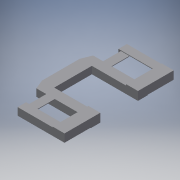
# Autodesk Inventor part: battlebotupperframe
Saved by Autodesk Inventor 2019 (Build 230136000, 136)
## iProperties
Created: 2018-08-05
Part Number: battlebotupperframe
Material: Generic
Document SubType Name: Modeling
Designer: Kitte_X
Density: 1 g/cm^3
Appearance: Default
Author: Kitte_X
Autodesk Inventor part; units mm, degrees
ref_plane "YZ Plane" through (0, 0, 0) normal (1, 0, 0) x (0, 1, 0)
ref_plane "XZ Plane" through (0, 0, 0) normal (0, 1, 0) x (-1, 0, 0)
ref_plane "XY Plane" through (0, 0, 0) normal (0, 0, 1) x (1, 0, 0)
sketch "Sketch1" plane through (0, 0, 0) normal (0, 1, 0) x (-1, 0, 0)
  line L0 (-100, 284.5) -> (-100, 98)
  line L1 (-100, 98) -> (140, 98)
  line L2 (140, 98) -> (140, -98)
  line L3 (140, -98) -> (-100, -98)
  line L4 (-100, -98) -> (-100, -284.5)
  line L5 (-100, 284.5) -> (144, 284.5)
  line L6 (144, 284.5) -> (144, 240.5)
  line L7 (144, 240.5) -> (131.5, 240.5)
  line L8 (131.5, 240.5) -> (131.5, 148)
  line L9 (131.5, 148) -> (183.5, 148)
  line L10 (183.5, 148) -> (203.5, 98)
  line L11 (-100, -284.5) -> (144, -284.5)
  line L12 (144, -284.5) -> (144, -240.5)
  line L13 (144, -240.5) -> (131.5, -240.5)
  line L14 (131.5, -240.5) -> (131.5, -148)
  line L15 (131.5, -148) -> (183.5, -148)
  line L16 (183.5, -148) -> (203.5, -98)
  line L17 (203.5, 98) -> (203.5, -98)
  line L18 (-38, 240.5) -> (-38, 148)
  line L19 (-38, 148) -> (87, 148)
  line L20 (87, 148) -> (87, 240.5)
  line L21 (87, 240.5) -> (-38, 240.5)
  line L22 (-38, -148) -> (-38, -240.5)
  line L23 (-38, -240.5) -> (87, -240.5)
  line L24 (87, -240.5) -> (87, -148)
  line L25 (87, -148) -> (-38, -148)
  point P0 (0, 0)
  point P1 (140, 0)
  dimension "d4" = 196
  dimension "d8" = 244
  dimension "d9" = 44
  dimension "d10" = 12.5
  dimension "d12" = 52
  dimension "d13" = 50
  dimension "d14" = 20
  dimension "d17" = 12.5
  dimension "d19" = 52
  dimension "d20" = 50
  dimension "d21" = 20
  dimension "d23" = 92.5
  dimension "d24" = 125
  dimension "d25" = 62
  dimension "d26" = 44
  dimension "d27" = 92.5
  dimension "d28" = 125
  dimension "d29" = 62
  dimension "d30" = 44
  dimension "d64" = 240
  dimension "d65" = 240
  dimension "d66" = 50
  dimension "d69" = 92.5
  dimension "d70" = 196
  dimension "d76" = 44
  constraints: 53 end point, 16 perpendicular, 6 point on line, 3 horizontal, 3 vertical, 1 horizontal alignment, 1 midpoint
  measures "d4" distance of L1.end L2.end
  measures "d8" distance of L0.start L5.end
  measures "d9" distance of L5.end L6.end
  measures "d10" distance of L6.end L7.end
  measures "d12" distance of L8.end L9.end
  measures "d13" vertical distance of L9.end L10.end
  measures "d14" horizontal distance of L9.end L10.end
  measures "d17" distance of L12.end L13.end
  measures "d19" distance of L14.end L15.end
  measures "d20" vertical distance of L15.end L16.end
  measures "d21" horizontal distance of L15.end L16.end
  measures "d23" distance of L18.start L18.end
  measures "d24" distance of L18.end L19.end
  measures "d25" distance between parallel lines of L0 L18
  measures "d26" distance between parallel lines of L5 L21
  measures "d27" distance of L22.start L22.end
  measures "d28" distance of L22.end L23.end
  measures "d29" distance between parallel lines of L4 L22
  measures "d30" distance between parallel lines of L11 L23
  measures "d64" distance of L0.end L1.end
  measures "d65" distance of L2.end L3.end
  measures "d66" distance between parallel lines of L3 L25
  measures "d69" distance of L7.end L8.end
  measures "d70" distance of L10.end L16.end
  measures "d76" distance of L11.end L12.end
extrude "Extrusion1" add sketch "Sketch1" along normal blind 6.5
sketch "Sketch3" plane through (0, 0, 0) normal (0, -1, 0) x (1, 0, 0)
  line L0 (-87, -148) -> (38, -148) construction
  line L1 (38, -148) -> (38, -240.5) construction
  line L2 (38, -240.5) -> (-87, -240.5) construction
  line L3 (-87, -240.5) -> (-87, -148) construction
  line L4 (-87, 240.5) -> (38, 240.5) construction
  line L5 (38, 240.5) -> (38, 148) construction
  line L6 (38, 148) -> (-87, 148) construction
  line L7 (-87, 148) -> (-87, 240.5) construction
  line L8 (100, 284.5) -> (100, 98) construction
  line L9 (-144, 284.5) -> (100, 284.5) construction
  line L10 (-144, 240.5) -> (-144, 284.5) construction
  line L11 (-131.5, 240.5) -> (-144, 240.5) construction
  line L12 (-131.5, 148) -> (-131.5, 240.5) construction
  line L13 (-183.5, 148) -> (-131.5, 148) construction
  line L14 (-203.5, 98) -> (-183.5, 148) construction
  line L15 (-203.5, -98) -> (-203.5, 98) construction
  line L16 (-183.5, -148) -> (-203.5, -98) construction
  line L17 (-131.5, -148) -> (-183.5, -148) construction
  line L18 (-131.5, -240.5) -> (-131.5, -148) construction
  line L19 (-144, -240.5) -> (-131.5, -240.5) construction
  line L20 (-144, -284.5) -> (-144, -240.5) construction
  line L21 (100, -284.5) -> (-144, -284.5) construction
  line L22 (100, -98) -> (100, -284.5) construction
  line L23 (-140, -98) -> (100, -98) construction
  line L24 (-140, 98) -> (-140, -98) construction
  line L25 (100, 98) -> (-140, 98) construction
  line L26 (100, -98) -> (100, -284.5) projected
  line L27 (-131.5, -148) -> (-183.5, -148) projected
  line L28 (100, -98) -> (-203.5, -98)
  line L29 (-140, -98) -> (100, -98) projected
  line L30 (-183.5, -148) -> (-203.5, -98) projected
  line L31 (-183.5, -148) -> (100, -148)
  line L32 (100, -98) -> (100, -284.5) projected
  line L33 (100, -98) -> (100, -148)
  line L34 (100, 284.5) -> (100, 98) projected
  line L35 (-203.5, -98) -> (-203.5, 98) projected
  line L36 (100, 98) -> (-203.5, 98)
  line L37 (-203.5, 98) -> (-183.5, 148)
  line L38 (100, 148) -> (100, 98)
  line L39 (-183.5, 148) -> (-131.5, 148) projected
  line L40 (100, 148) -> (-183.5, 148)
  line L41 (-183.5, -148) -> (-203.5, -98)
  line L42 (-203.5, -98) -> (-183.5, -148)
  point P0 (0, 0)
  constraints: 18 end point, 6 collinear, 2 point on line, 1 horizontal, 1 parallel
extrude "Extrusion3" add sketch "Sketch3" along normal blind 38
sketch "Sketch4" plane through (0, 0, 0) normal (0, -1, 0) x (1, 0, 0)
  line L0 (-203.5, -98) -> (-203.5, 98) projected
  line L1 (-140, 98) -> (-203.5, 98) projected
  line L2 (-203.5, 98) -> (-140, 98)
  line L3 (-140, 98) -> (-140, -98) projected
  line L4 (-140, 98) -> (-140, -98)
  line L5 (-140, -98) -> (-203.5, -98)
  line L6 (-203.5, -98) -> (-203.5, 98)
  point P0 (0, 0)
  constraints: 8 end point, 2 collinear, 2 perpendicular
extrude "Extrusion4" add sketch "Sketch4" along normal blind 38
sketch "Sketch5" plane through (0, 6.5, 0) normal (0, 1, 0) x (1, 0, 0)
  line L0 (38, 148) -> (-87, 148) construction
  line L1 (-87, 148) -> (-87, 240.5) construction
  line L2 (-87, 240.5) -> (38, 240.5) construction
  line L3 (38, 240.5) -> (38, 148) construction
  line L4 (38, -240.5) -> (-87, -240.5) construction
  line L5 (-87, -240.5) -> (-87, -148) construction
  line L6 (-87, -148) -> (38, -148) construction
  line L7 (38, -148) -> (38, -240.5) construction
  line L8 (100, -284.5) -> (100, -98) construction
  line L9 (100, -98) -> (-140, -98) construction
  line L10 (-140, -98) -> (-140, 98) construction
  line L11 (-140, 98) -> (100, 98) construction
  line L12 (100, 98) -> (100, 284.5) construction
  line L13 (100, 284.5) -> (-144, 284.5) construction
  line L14 (-144, 284.5) -> (-144, 240.5) construction
  line L15 (-144, 240.5) -> (-131.5, 240.5) construction
  line L16 (-131.5, 240.5) -> (-131.5, 148) construction
  line L17 (-131.5, 148) -> (-183.5, 148) construction
  line L18 (-183.5, 148) -> (-203.5, 98) construction
  line L19 (-203.5, 98) -> (-203.5, -98) construction
  line L20 (-203.5, -98) -> (-183.5, -148) construction
  line L21 (-183.5, -148) -> (-131.5, -148) construction
  line L22 (-131.5, -148) -> (-131.5, -240.5) construction
  line L23 (-131.5, -240.5) -> (-144, -240.5) construction
  line L24 (-144, -240.5) -> (-144, -284.5) construction
  line L25 (-144, -284.5) -> (100, -284.5) construction
  line L26 (-140, -98) -> (-140, 98) projected
  line L27 (-140, -98) -> (-140, 98)
  line L28 (-140, 98) -> (100, 98) projected
  line L29 (-140, 98) -> (38, 98)
  line L30 (38, 240.5) -> (38, 148) projected
  line L31 (38, 98) -> (38, 148)
  line L32 (-87, 240.5) -> (-87, 148) projected
  line L33 (-87, 148) -> (-87, 240.5)
  line L34 (-131.5, 240.5) -> (-131.5, 148) projected
  line L35 (-131.5, 148) -> (-131.5, 240.5)
  line L36 (38, 148) -> (-87, 148) projected
  line L37 (38, 148) -> (-87, 148)
  line L38 (-131.5, 148) -> (-183.5, 148) projected
  line L39 (-131.5, 148) -> (-183.5, 148)
  line L40 (-183.5, 148) -> (-203.5, 98)
  line L41 (-203.5, 98) -> (-203.5, -98) projected
  line L42 (-203.5, 98) -> (-203.5, -98)
  line L43 (100, -148) -> (-183.5, -148) projected
  line L44 (-203.5, -98) -> (-183.5, -148)
  line L45 (-183.5, -148) -> (-131.5, -148)
  line L46 (-131.5, -148) -> (-131.5, -240.5) projected
  line L47 (-131.5, -148) -> (-131.5, -240.5)
  line L48 (-87, -240.5) -> (-87, -148) projected
  line L49 (-87, -240.5) -> (-87, -148)
  line L50 (-87, -148) -> (38, -148)
  line L51 (-140, -98) -> (100, -98) projected
  line L52 (38, -98) -> (38, -148)
  line L53 (38, -98) -> (-140, -98)
  line L54 (38, -148) -> (38, -240.5) projected
  line L55 (38, -240.5) -> (38, -284.5)
  line L56 (-144, -284.5) -> (100, -284.5) projected
  line L57 (-144, -240.5) -> (-144, -284.5) projected
  line L58 (-144, -284.5) -> (-144, -240.5)
  line L59 (-144, -240.5) -> (-131.5, -240.5)
  line L60 (38, -240.5) -> (-87, -240.5) projected
  line L61 (-87, -240.5) -> (38, -240.5)
  line L62 (38, -284.5) -> (-144, -284.5)
  line L63 (38, 240.5) -> (-87, 240.5) projected
  line L64 (-87, 240.5) -> (38, 240.5)
  line L65 (38, 240.5) -> (38, 284.5)
  line L66 (100, 284.5) -> (-144, 284.5) projected
  line L67 (-144, 284.5) -> (38, 284.5)
  line L68 (-144, 284.5) -> (-144, 240.5) projected
  line L69 (-144, 284.5) -> (-144, 240.5)
  line L70 (-144, 240.5) -> (-131.5, 240.5)
  point P0 (0, 0)
  constraints: 52 end point, 17 collinear, 5 perpendicular, 5 point on line, 1 vertical
extrude "Extrusion5" cut sketch "Sketch5" against normal blind 3.25 contours L51 L52 L43 L44 L41 L40 L38 L34 L70 L68 L66 L65 L63 L32 L36 L31 L28 L26 | L48 L60 L55 L56 L57 L59 L46 L43
sketch "Sketch6" plane through (0, 3.25, 0) normal (0, 1, 0) x (1, 0, 0)
  line L0 (-87, 148) -> (38, 148) construction
  line L1 (-87, 240.5) -> (-87, 148) construction
  line L2 (38, 240.5) -> (-87, 240.5) construction
  line L3 (38, 284.5) -> (38, 240.5) construction
  line L4 (-144, 284.5) -> (38, 284.5) construction
  line L5 (-144, 240.5) -> (-144, 284.5) construction
  line L6 (-131.5, 240.5) -> (-144, 240.5) construction
  line L7 (-131.5, 148) -> (-131.5, 240.5) construction
  line L8 (-183.5, 148) -> (-131.5, 148) construction
  line L9 (-203.5, 98) -> (-183.5, 148) construction
  line L10 (-203.5, -98) -> (-203.5, 98) construction
  line L11 (-183.5, -148) -> (-203.5, -98) construction
  line L12 (-131.5, -148) -> (-183.5, -148) construction
  line L13 (-131.5, -240.5) -> (-131.5, -148) construction
  line L14 (-144, -240.5) -> (-131.5, -240.5) construction
  line L15 (-144, -284.5) -> (-144, -240.5) construction
  line L16 (38, -284.5) -> (-144, -284.5) construction
  line L17 (38, -240.5) -> (38, -284.5) construction
  line L18 (-87, -240.5) -> (38, -240.5) construction
  line L19 (-87, -148) -> (-87, -240.5) construction
  line L20 (38, -148) -> (-87, -148) construction
  line L21 (38, -98) -> (38, -148) construction
  line L22 (-140, -98) -> (38, -98) construction
  line L23 (-140, 98) -> (-140, -98) construction
  line L24 (38, 98) -> (-140, 98) construction
  line L25 (38, 148) -> (38, 98) construction
  line L26 (38, -149) -> (-87, -149) projected
  line L27 (38, -148) -> (-87, -148)
  line L28 (-87, -148) -> (-87, -240.5)
  line L29 (-131.5, -240.5) -> (-87, -240.5)
  line L30 (-131.5, -148) -> (-131.5, -240.5) projected
  line L31 (-131.5, -240.5) -> (-131.5, -148)
  line L32 (100, -148) -> (-183.5, -148) projected
  line L33 (-131.5, -148) -> (-183.5, -148)
  line L34 (-203.5, -98) -> (-203.5, 98) projected
  line L35 (-183.5, -148) -> (-203.5, -98)
  line L36 (-203.5, -98) -> (-203.5, 98)
  line L37 (-203.5, 98) -> (-183.5, 148)
  line L38 (-131.5, 240.5) -> (-131.5, 148) projected
  line L39 (-183.5, 148) -> (100, 148) projected
  line L40 (-131.5, 148) -> (-183.5, 148)
  line L41 (-144, 240.5) -> (-131.5, 240.5) projected
  line L42 (-131.5, 148) -> (-131.5, 240.5)
  line L43 (-131.5, 240.5) -> (-87, 240.5)
  line L44 (-87, 240.5) -> (-87, 148) projected
  line L45 (-87, 148) -> (-87, 240.5)
  line L46 (38, 148) -> (38, 240.5) projected
  line L47 (-87, 148) -> (38, 148)
  line L48 (38, 148) -> (38, 98) projected
  line L49 (38, 148) -> (38, 98)
  line L50 (100, 98) -> (-140, 98) projected
  line L51 (38, 98) -> (-140, 98)
  line L52 (-140, 98) -> (-140, -98) projected
  line L53 (-140, 98) -> (-140, -98)
  line L54 (-140, -98) -> (38, -98)
  line L55 (38, -98) -> (38, -284.5) projected
  line L56 (38, -148) -> (38, -98)
  point P0 (0, 0)
  constraints: 36 end point, 6 perpendicular, 5 collinear, 2 horizontal, 2 vertical, 1 parallel
extrude "Extrusion6" add sketch "Sketch6" against normal blind 6.25 contours L28 L29 L30 L32 | L27 L32 L35 L34 L37 L39 L48 L50 L52 L54 L55 | L39 L38 L43 L44
extrude "Extrusion7" cut sketch "Sketch6" against normal blind 3.25 contours L28 L29 L30 L32 | L27 L32 L35 L34 L37 L39 L48 L50 L52 L54 L55 | L39 L38 L43 L44
sketch "Sketch7" plane through (0, 0, 0) normal (0, -1, 0) x (1, 0, 0)
  line L0 (38, 148) -> (100, 148) projected
  line L1 (93.5, 148) -> (100, 148)
  line L2 (100, 284.5) -> (100, 148) projected
  line L3 (100, 285) -> (100, 148)
  line L4 (-144, 284.5) -> (100, 284.5) projected
  line L5 (-144, 240.5) -> (-144, 284.5) projected
  line L6 (100, 284.5) -> (-144, 284.5)
  line L7 (-144, 240.5) -> (-144, 284.5)
  line L8 (93.5, 280) -> (93.5, 148)
  line L9 (-144, 240.5) -> (38, 240.5) projected
  line L10 (-141, 240.5) -> (-141, 280)
  line L11 (-141, 280) -> (93.5, 280)
  line L12 (-141, 240.5) -> (-144, 240.5)
  line L13 (-573.3935, 0) -> (506.825, 0) construction
  line L14 (93.5, -148) -> (100, -148)
  line L15 (100, -284.5) -> (100, -148)
  line L16 (-144, -284.5) -> (100, -284.5)
  line L17 (-144, -240.5) -> (-144, -284.5)
  line L18 (100, -284.5) -> (-144, -284.5)
  line L19 (93.5, -280) -> (93.5, -148)
  line L20 (-141, -240.5) -> (-141, -280)
  line L21 (38, -240.5) -> (38, -148) construction
  line L22 (38, -240.5) -> (-144, -240.5) construction
  line L23 (-141, -240.5) -> (-144, -240.5)
  line L24 (-141, -280) -> (93.5, -280)
  line L25 (-144, -240.5) -> (-144, -284.5) projected
  line L26 (100, -98) -> (100, -284.5) projected
  line L27 (100, -148) -> (100, -284.5)
  point P0 (0, 0)
  dimension "d85" = 3
  dimension "d86" = 4.5
  dimension "d87" = 6.5
  constraints: 40 end point, 10 symmetric about line, 4 collinear, 4 perpendicular, 3 point on line, 2 horizontal, 2 vertical, 1 parallel
  measures "d85" distance between parallel lines of L5 L10
  measures "d86" distance between parallel lines of L4 L11
  measures "d87" distance between parallel lines of L3 L8
extrude "Extrusion8" add sketch "Sketch7" along normal blind 35.5
sketch "Sketch8" plane through (100, 6.5, 284.5) normal (1, 0, 0) x (0, 0, -1)
  line L0 (142.5, -38.5) -> (142.5, -12.5)
  line L1 (142.5, -12.5) -> (180.5, -12.5)
  line L2 (180.5, -38.5) -> (142.5, -38.5)
  line L3 (180.5, -12.5) -> (180.5, -38.5)
  line L4 (186.5, -44.5) -> (186.5, 0) projected
  line L5 (186.5, -44.5) -> (136.5, -44.5) projected
  line L6 (136.5, -42) -> (136.5, -44.5) projected
  line L7 (0, 0) -> (186.5, 0) projected
  line L8 (285, -82.0279) -> (285, 56.7605) construction
  line L9 (427.5, -38.5) -> (427.5, -12.5)
  line L10 (427.5, -12.5) -> (389.5, -12.5)
  line L11 (389.5, -38.5) -> (427.5, -38.5)
  line L12 (389.5, -12.5) -> (389.5, -38.5)
  point P0 (284.5, -6.5)
  point P1 (136.5, -6.5)
  dimension "d90" = 6
  dimension "d91" = 6
  dimension "d92" = 6
  dimension "d93" = 12.5
  constraints: 18 end point, 4 symmetric about line, 3 vertical, 1 parallel
  measures "d90" distance between parallel lines of L4 L3
  measures "d91" distance between parallel lines of L5 L2
  measures "d92" distance between parallel lines of L0 L6
  measures "d93" distance between parallel lines of L7 L1
extrude "Extrusion9" cut sketch "Sketch8" against normal through all
extrude "Extrusion10" add sketch "Sketch8" against normal blind 6.5
body "Solid1"
